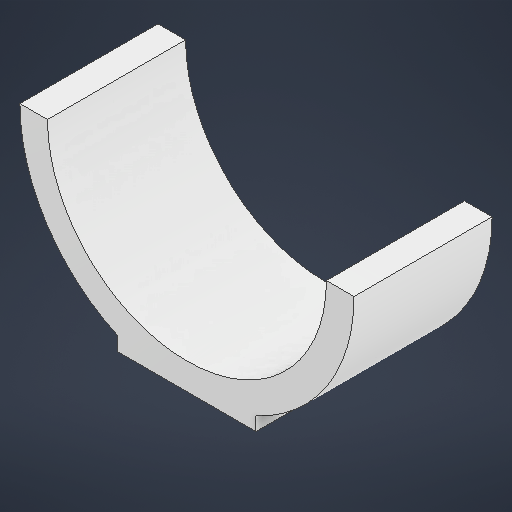
# Autodesk Inventor part: clip-pipe
Saved by Autodesk Inventor 2025.2 (Build 292293000, 293)
## iProperties
Created: 2026-01-03
Part Number: clip-pipe
Material: PC/ABS Plastic
Document SubType Name: Modeling
Designer: sam
Density: 1.1 g/cm^3
Appearance: Smooth - White
Author: sam
Autodesk Inventor part; units mm, degrees
ref_plane "YZ Plane" through (0, 0, 0) normal (1, 0, 0) x (0, 1, 0)
ref_plane "XZ Plane" through (0, 0, 0) normal (0, 1, 0) x (-1, 0, 0)
ref_plane "XY Plane" through (0, 0, 0) normal (0, 0, 1) x (1, 0, 0)
sketch "Sketch2" plane through (0, 0, 0) normal (0, 0, 1) x (1, 0, 0)
  circle A0 centre (3.2039, 2.261) radius 12.1
  circle A1 centre (3.2039, 2.261) radius 10.1
  line L0 (-1.7961, -8.7576) -> (8.2039, -8.7576)
  line L1 (-1.7961, -8.7576) -> (-1.7961, -9.7576)
  line L2 (-1.7961, -9.7576) -> (8.2039, -9.7576)
  line L3 (8.2039, -9.7576) -> (8.2039, -8.7576)
  line L4 (-6.8961, 2.261) -> (-8.8961, 2.261)
  line L5 (13.3039, 2.261) -> (15.3039, 2.261)
  dimension "d6" = 24.2
  dimension "d7" = 20.2
  dimension "d8" = 1
  dimension "d9" = 10
  constraints: 12 end point, 6 point on circle, 2 centre point, 2 horizontal, 2 perpendicular, 2 point on line, 1 coincident, 1 vertical
  measures "d6" diameter of A0
  measures "d7" diameter of A1
  measures "d8" distance of L0.start L1.end
  measures "d9" distance of L0.start L0.end
extrude "Extrusion2" add sketch "Sketch2" along normal blind 10 contours A0 L0 L4 A1 L5 | L3 L2 A0 | A0 L2 L0 | A0 L2 L1
body "Solid2"
